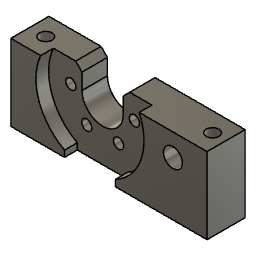
Trident M1 rev1 Mount2 (Autodesk Fusion 360 archive; units mm, degrees)
design "Mount v1"
Autodesk Fusion 360 part; units mm, degrees
sketch "スケッチ1" plane through (0, 0, 0) normal (0, 0, 1) x (1, 0, 0)
  line L0 (0, 0) -> (30, 0)
  line L1 (30, 0) -> (30, 17)
  line L2 (30, 17) -> (0, 17)
  line L3 (0, 17) -> (0, 0)
  dimension "d1" = 30
  dimension "d2" = 17
  constraint horizontal L0
  constraint vertical L1
  constraint horizontal L2
  constraint vertical L3
  constraint coincident L0.start L3.end
  measures "d1" distance of L0.start L0.end
  measures "d2" distance of L0.start L2.end
extrude "押し出し1" add sketch "スケッチ1" along normal blind 6
sketch "スケッチ2" plane through (0, 0, 0) normal (0, -1, 0) x (1, 0, 0)
  line L0 (0, 0) -> (30, 0)
  line L1 (30, 0) -> (30, 6)
  line L2 (30, 6) -> (0, 6)
  line L3 (0, 6) -> (0, 0)
  line L4 (30, 0) -> (30, 3)
  circle A0 centre (28.25, 3) radius 1
  circle A1 centre (2, 3) radius 1
  dimension "d7" = 2
  dimension "d9" = 2
  constraint coincident L0.end L1.start
  constraint midpoint L1 L4.end
  measures "d7" diameter of A0
  measures "d9" diameter of A1
extrude "押し出し2" cut sketch "スケッチ2" against normal blind 100 contours A0 | A1
sketch "スケッチ3" plane through (0, 0, 6) normal (0, 0, 1) x (1, 0, 0)
  line L0 (0, 17) -> (0, 0)
  line L1 (0, 0) -> (30, 0)
  line L2 (30, 0) -> (30, 17)
  line L3 (30, 17) -> (0, 17)
  line L4 (30, 17) -> (25, 17)
  line L5 (25, 0) -> (25, 7)
  line L6 (26.5, 8.5) -> (30, 8.5)
  circle A0 centre (25, 8.5) radius 1.5
  line L7 (25, 17) -> (25, 10)
  line L8 (25, 7) -> (25, 0)
  line L9 (25, 8.5) -> (11.95, 8.5)
  circle A1 centre (11.95, 8.5) radius 8.5
  circle A2 centre (16.95, 8.5) radius 0.805
  circle A3 centre (14.45, 12.8301) radius 0.805
  circle A4 centre (9.45, 12.8301) radius 0.805
  circle A5 centre (6.95, 8.5) radius 0.805
  circle A6 centre (9.45, 4.1699) radius 0.805
  circle A7 centre (14.45, 4.1699) radius 0.805
  circle A8 centre (11.95, 8.5) radius 3.25
  dimension "d12" = 3
  dimension "d13" = 13.05
  dimension "d15" = 1.61
  dimension "d17" = 360
  dimension "d18" = 6.5
  constraint coincident L2.end L3.start
  constraint coincident L3 L4.end
  constraint perpendicular L2 L4
  constraint coincident L1 L5.start
  constraint perpendicular L1 L7
  constraint midpoint L2 L6.end
  constraint coincident A0 L6.start
  constraint coincident A0 L7.end
  constraint coincident A0 L5.end
  constraint collinear L7 L8
  constraint coincident A0.centre L9.start
  constraint parallel L3 L9
  constraint coincident L9.end A1.centre
  constraint tangent L1 A1
  constraint coincident L9 A2.centre
  constraint concentric A1 A8
  measures "d12" diameter of A0
  measures "d13" distance of A0.centre L9.end
  measures "d15" diameter of A2
  measures "d18" diameter of A8
extrude "押し出し3" cut sketch "スケッチ3" against normal blind 10 contours A0 | L9 A2 | L9 A2 | A3 | A4 | A5 | A6 | A7 | A8
extrude "押し出し4" cut sketch "スケッチ3" against normal blind 1 contours A1
sketch "スケッチ4" plane through (0, 0, 6) normal (0, 0, 1) x (1, 0, 0)
  arc A0 (11.95, 17) -> (11.95, 0) centre (11.95, 8.5) ccw
  line L0 (11.95, 17) -> (0, 17)
  line L1 (0, 17) -> (0, 0)
  line L2 (0, 0) -> (11.95, 0)
  line L3 (11.95, 8.5) -> (11.95, 1)
  line L4 (11.95, 1) -> (7.95, 1)
  line L5 (11.95, 1) -> (15.95, 1)
  line L6 (7.95, 1) -> (7.95, 0)
  line L7 (15.95, 1) -> (15.95, 0)
  line L8 (15.95, 0) -> (7.95, 0)
  dimension "d23" = 1
  dimension "d24" = 4
  constraint coincident A0.centre L3.start
  constraint coincident A0 L4.end
  constraint perpendicular L3 L4
  constraint coincident L2 L6.end
  constraint perpendicular L2 L6
  constraint perpendicular L5 L7
  constraint perpendicular L6 L8
  measures "d23" distance of A0.end L3.end
  measures "d24" distance of L3.end L5.end
extrude "押し出し5" cut sketch "スケッチ4" against normal blind 1 contours A0 L4 L5 L7 L8 | A0 L2 L6 L8
sketch "スケッチ5" plane through (0, 0, 6) normal (0, 0, 1) x (1, 0, 0)
  line L0 (15.95, 1) -> (15.95, 0)
  line L1 (15.95, 0) -> (30, 0)
  line L2 (30, 0) -> (30, 17)
  line L3 (30, 17) -> (11.95, 17)
  arc A0 (15.95, 1) -> (11.95, 17) centre (11.95, 8.5) ccw
  circle A1 centre (25, 8.5) radius 1.5
  line L4 (26.6454, 5.65) -> (28.2909, 8.5)
  line L5 (28.2909, 8.5) -> (26.6454, 11.35)
  line L6 (26.6454, 11.35) -> (23.3546, 11.35)
  line L7 (23.3546, 11.35) -> (21.7091, 8.5)
  line L8 (21.7091, 8.5) -> (23.3546, 5.65)
  line L9 (23.3546, 5.65) -> (26.6454, 5.65)
  point P0 (25, 8.5)
  point P1 (25, 8.5)
  dimension "d60" = 2.85
  constraint coincident P1 P0
  measures "d60" distance of P1 L9
extrude "押し出し6" cut sketch "スケッチ5" against normal blind 1.5 contours L4 L5 L6 L7 L8 L9
sketch "スケッチ6" plane through (30, 0, 0) normal (1, 0, 0) x (0, 0, -1)
  line L0 (0, 0) -> (0, 17)
  line L1 (0, 17) -> (-6, 17)
  line L2 (-6, 17) -> (-6, 0)
  line L3 (-6, 0) -> (0, 0)
  line L4 (-6, 0) -> (0, 0)
  line L5 (0, 0) -> (0, 12)
  line L6 (0, 12) -> (-6, 12)
  line L7 (-6, 12) -> (-6, 0)
  dimension "d30" = 6
  dimension "d31" = 12
  constraint horizontal L4
  constraint vertical L5
  constraint horizontal L6
  constraint vertical L7
  constraint coincident L2.end L3.start
  measures "d30" distance of L2.end L0.start
  measures "d31" distance of L2.end L6.end
extrude "押し出し7" cut sketch "スケッチ6" against normal blind 100 contours L0 L1 L2 L6
sketch "スケッチ7" plane through (0, 0, 0) normal (0, 0, -1) x (-1, 0, 0)
  line L0 (0, 12) -> (-30, 12)
  line L1 (-30, 12) -> (-30, 0)
  line L2 (-30, 0) -> (0, 0)
  line L3 (0, 0) -> (0, 12)
  circle A0 centre (-11.95, 8.5) radius 3.25
  circle A1 centre (-25, 8.5) radius 1.5
  circle A2 centre (-6.95, 8.5) radius 0.805
  circle A3 centre (-14.45, 4.1699) radius 0.805
  circle A4 centre (-16.95, 8.5) radius 0.805
  circle A5 centre (-9.45, 4.1699) radius 0.805
  line L4 (-11.95, 8.5) -> (-8.7, 8.5)
  line L5 (-8.7, 8.5) -> (-8.7, 12)
  line L6 (-11.95, 8.5) -> (-15.2, 8.5)
  line L7 (-15.2, 8.5) -> (-15.2, 12)
  line L8 (-15.2, 12) -> (-8.7, 12)
  constraint coincident A0.centre L4.start
  constraint coincident A0 L4.end
  constraint parallel L0 L4
  constraint coincident L0 L5.end
  constraint tangent A0 L5
  constraint coincident A0 L6.end
  constraint perpendicular L5 L6
  constraint coincident L0 L7.end
  constraint tangent A0 L7
extrude "押し出し8" cut sketch "スケッチ7" against normal blind 10 contours L0 A0 L5 L7 L8
sketch "スケッチ8" plane through (0, 12, 0) normal (0, 1, 0) x (-1, 0, 0)
  line L0 (-15.2, 0) -> (-15.2, 5)
  line L1 (-15.2, 5) -> (-19.696, 5)
  line L2 (-19.696, 5) -> (-19.696, 6)
  line L3 (-19.696, 6) -> (-30, 6)
  line L4 (-30, 6) -> (-30, 0)
  line L5 (-30, 0) -> (-15.2, 0)
  circle A0 centre (-28.25, 3) radius 1
  line L6 (-26.15, 4.2124) -> (-28.25, 5.4249)
  line L7 (-28.25, 5.4249) -> (-30.35, 4.2124)
  line L8 (-30.35, 4.2124) -> (-30.35, 1.7876)
  line L9 (-30.35, 1.7876) -> (-28.25, 0.5751)
  line L10 (-28.25, 0.5751) -> (-26.15, 1.7876)
  line L11 (-26.15, 1.7876) -> (-26.15, 4.2124)
  point P0 (-28.25, 3)
  dimension "d36" = 2.1
  constraint coincident P0 A0.centre
  measures "d36" distance of P0 L11
extrude "押し出し9" cut sketch "スケッチ8" against normal blind 0.5 contours L4 L6 L7 L9 L10 L11
sketch "スケッチ9" plane through (0, 12, 0) normal (0, 1, 0) x (-1, 0, 0)
  line L0 (-8.7, 5) -> (-8.7, 0)
  line L1 (-8.7, 0) -> (0, 0)
  line L2 (0, 0) -> (0, 6)
  line L3 (0, 6) -> (-4.204, 6)
  line L4 (-4.204, 6) -> (-4.204, 5)
  line L5 (-4.204, 5) -> (-8.7, 5)
  circle A0 centre (-2, 3) radius 1
  line L6 (-4.1009, 1.789) -> (-2.0017, 0.5751)
  line L7 (-2.0017, 0.5751) -> (0.0991, 1.7861)
  line L8 (0.0991, 1.7861) -> (0.1009, 4.211)
  line L9 (0.1009, 4.211) -> (-1.9983, 5.4249)
  line L10 (-1.9983, 5.4249) -> (-4.0991, 4.2139)
  line L11 (-4.0991, 4.2139) -> (-4.1009, 1.789)
  point P0 (-2, 3)
  dimension "d39" = 2.1
  constraint coincident P0 A0.centre
  measures "d39" distance of P0 L11
extrude "押し出し10" cut sketch "スケッチ9" against normal blind 0.5 contours L2 L6 L7 L9 L10 L11
extrude "押し出し11" add 1 faces at (30, 3.8333, 2.5285) along direction (1, 0, 0) blind 0.375
extrude "押し出し12" add 1 faces at (30, 11.5, 3) along direction (0, 1, 0) blind 0.5
sketch "スケッチ10" plane through (0, 12, 0) normal (0, 1, 0) x (-1, 0, 0)
  line L0 (-30.375, 6) -> (-30.375, 0)
  line L1 (-30.375, 0) -> (-15.2, 0)
  line L2 (-15.2, 0) -> (-15.2, 5)
  line L3 (-15.2, 5) -> (-19.696, 5)
  line L4 (-19.696, 5) -> (-19.696, 6)
  line L5 (-19.696, 6) -> (-30.375, 6)
  circle A0 centre (-28.25, 3) radius 1
  line L6 (-30.5687, 1.705) -> (-28.2878, 0.3445)
  line L7 (-28.2878, 0.3445) -> (-25.9691, 1.6395)
  line L8 (-25.9691, 1.6395) -> (-25.9313, 4.295)
  line L9 (-25.9313, 4.295) -> (-28.2122, 5.6555)
  line L10 (-28.2122, 5.6555) -> (-30.5309, 4.3605)
  line L11 (-30.5309, 4.3605) -> (-30.5687, 1.705)
  point P0 (-28.25, 3)
  point P1 (-28.25, 3)
  dimension "d61" = 2.3
  constraint coincident P1 P0
  measures "d61" distance of P1 L11
extrude "押し出し13" cut sketch "スケッチ10" against normal blind 0.5 contours L0 L6 L7 L8 L9 L10
extrude "押し出し15" add 1 faces at (0, 3.8333, 3.4231) along direction (-1, 0, 0) blind 0.5
extrude "押し出し16" add 1 faces at (0, 11.5, 2.9994) along direction (0, 1, 0) blind 0.5
sketch "スケッチ11" plane through (0, 12, 0) normal (0, 1, 0) x (-1, 0, 0)
  line L0 (0.5, 0) -> (0.5, 6)
  line L1 (0.5, 6) -> (-4.204, 6)
  line L2 (-4.204, 6) -> (-4.204, 5)
  line L3 (-4.204, 5) -> (-8.7, 5)
  line L4 (-8.7, 5) -> (-8.7, 0)
  line L5 (-8.7, 0) -> (0.5, 0)
  circle A0 centre (-2, 3) radius 1
  line L6 (0.3, 4.3279) -> (-2, 5.6558)
  line L7 (-2, 5.6558) -> (-4.3, 4.3279)
  line L8 (-4.3, 4.3279) -> (-4.3, 1.6721)
  line L9 (-4.3, 1.6721) -> (-2, 0.3442)
  line L10 (-2, 0.3442) -> (0.3, 1.6721)
  line L11 (0.3, 1.6721) -> (0.3, 4.3279)
  point P0 (-2, 3)
  dimension "d55" = 2.3
  constraint coincident P0 A0.centre
  measures "d55" distance of P0 L11
extrude "押し出し17" cut sketch "スケッチ11" against normal blind 0.5 contours L6 L7 L8 L9 L10 L11
extrude "押し出し18" cut 1 faces at (-0.3, 11.8333, 2.5574) along direction (-1, 0, 0) blind 10
chamfer "面取り1" distance 1 angle 45 1 edges at (15.2, 12, 2.5)
chamfer "面取り2" distance 1 angle 45 1 edges at (8.7, 12, 2.5)
extrude "押し出し19" add 1 faces at (3.8667, 11.5, 3) along direction (0, 1, 0) blind 0.5
extrude "押し出し20" add 1 faces at (27.3357, 11.5, 1.3726) along direction (0, 1, 0) blind 0.5
extrude "押し出し21" add 1 faces at (24.9626, 10.8986, 4.5) along direction (0, 0, 1) blind 1.5
extrude "押し出し22" cut 1 faces at (12.6492, 1.1576, 5) along direction (0, 0, -1) blind 1
